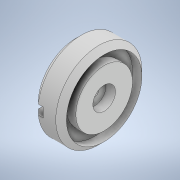
# Autodesk Inventor part: 711128
Saved by Autodesk Inventor 2022 (Build 260153000, 153)
## iProperties
Created: 2021-10-22
Part Number: 711128
Material: Типовые
Document SubType Name: Modeling
Designer: RaNSiD
Density: 1 g/cm^3
Appearance: По умолчанию
Mass: 19.6969 g
Surface Area: 64.5892 cm^2
Volume: 19.6969 cm^3
Author: RaNSiD
Autodesk Inventor part; units mm, degrees
ref_plane "YZ Plane" through (0, 0, 0) normal (1, 0, 0) x (0, 1, 0)
ref_plane "XZ Plane" through (0, 0, 0) normal (0, 1, 0) x (-1, 0, 0)
ref_plane "XY Plane" through (0, 0, 0) normal (0, 0, 1) x (1, 0, 0)
sketch "Эскиз1" plane through (0, 0, 0) normal (0, 0, 1) x (1, 0, 0)
  line L0 (0, 0) -> (0, 20)
  line L1 (0, 20) -> (2.8284, 22.8284)
  line L2 (0, 0) -> (15, 0)
  line L3 (15, 0) -> (15, 20)
  line L4 (15, 20) -> (12.1716, 22.8284)
  line L5 (12.1716, 22.8284) -> (2.8284, 22.8284)
  dimension "d0" = 20
  dimension "d1" = 4
  dimension "d2" = 135
  dimension "d3" = 15
  dimension "d4" = 4
  dimension "d5" = 135
  constraints: 12 end point, 1 horizontal, 1 parallel, 1 perpendicular, 1 vertical
  measures "d0" distance of L0.start L0.end
  measures "d1" distance of L0.end L1.end
  measures "d2" angle of L0 L1
  measures "d3" distance of L0.start L2.end
  measures "d4" distance of L3.end L4.end
  measures "d5" angle of L4 L3
revolve "Вращение1" add sketch "Эскиз1" angle 360 about axis through (0, 0, 0) along (1, 0, 0)
sketch "Эскиз2" plane through (0, 0, 0) normal (0, 0, 1) x (1, 0, 0)
  line L0 (15, -20) -> (15, 20) projected
  line L1 (15, 20) -> (10, 20)
  line L2 (10, 20) -> (10, 15)
  line L3 (10, 15) -> (15, 15)
  line L4 (15, 15) -> (15, 20)
  line L5 (15, 6) -> (10, 6)
  line L6 (10, 6) -> (10, 2)
  line L7 (10, 0) -> (15, 0)
  line L8 (15, 0) -> (15, 6)
  line L9 (10, 2) -> (6.8, 2)
  line L10 (6.8, 2) -> (6.8, 0)
  line L11 (6.8, 0) -> (10, 0)
  point P0 (0, 0)
  point P1 (15, 0)
  dimension "d7" = 5
  dimension "d8" = 5
  dimension "d9" = 6
  dimension "d10" = 2
  dimension "d11" = 5
  dimension "d12" = 3.2
  constraints: 22 end point, 5 parallel, 3 horizontal, 3 perpendicular, 2 horizontal alignment, 2 point on line, 1 midpoint, 1 vertical alignment
  measures "d7" distance of L3.end L2.end
  measures "d8" distance of L2.end L1.end
  measures "d9" distance between parallel lines of L7 L5
  measures "d10" distance between parallel lines of L11 L9
  measures "d11" distance of L5.start L5.end
  measures "d12" distance of L6.end L9.end
revolve "Вращение2" cut sketch "Эскиз2" angle 360 about axis through (6.8, 0, 0) along (1, 0, 0)
sketch "Эскиз4" plane through (0, 0, 0) normal (1, 0, 0) x (0, 1, 0)
  point P0 (0, 0)
  point P1 (17, 0)
  dimension "d17" = 17
  constraints: 1 horizontal alignment
  measures "d17" distance of point (0, 0) point (17, 0)
hole "Отверстие1" at (0, 17, 0) direction (1, 0, 0) diameter 3 depth 3 tip angle 90
sketch "Эскиз5" plane through (0, 0, 0) normal (0, 0, 1) x (1, 0, 0)
  line L0 (0, -20) -> (0, 20) projected
  line L1 (0, 2.5) -> (5.5, 2.5)
  line L2 (5.5, 2.5) -> (5.5, -2.5)
  line L3 (5.5, -2.5) -> (0, -2.5)
  line L4 (0, -2.5) -> (0, 2.5)
  point P0 (0, 0)
  point P1 (0, 0)
  point P2 (0, 0)
  dimension "d25" = 5
  dimension "d26" = 5.5
  constraints: 8 end point, 2 midpoint, 2 parallel, 1 coincident, 1 horizontal, 1 perpendicular, 1 point on line
  measures "d25" distance between parallel lines of L3 L1
  measures "d26" distance of L1.start L1.end
extrude "Выдавливание2" cut sketch "Эскиз5" along normal through all both and the other way through all
